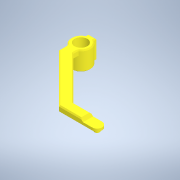
# Autodesk Inventor part: head_lock
Saved by Autodesk Inventor 2021 (Build 250183000, 183)
## iProperties
Created: 2021-02-04
Part Number: head_lock
Material: Generic
Document SubType Name: Modeling
Designer: Daniel
Density: 1 g/cm^3
Appearance: Default
Author: Daniel
Autodesk Inventor part; units mm, degrees
ref_plane "YZ Plane" through (0, 0, 0) normal (1, 0, 0) x (0, 1, 0)
ref_plane "XZ Plane" through (0, 0, 0) normal (0, 1, 0) x (-1, 0, 0)
ref_plane "XY Plane" through (0, 0, 0) normal (0, 0, 1) x (1, 0, 0)
sketch "Sketch1" plane through (0, 0, 0) normal (0, 1, 0) x (-1, 0, 0)
  arc A0 (-4.6069, -58.0567) -> (5, -60) centre (0, -60) ccw
  line L0 (0, 0) -> (-76, 0) construction
  line L1 (-5, -5) -> (-76, -5)
  line L2 (-76, 5) -> (5, 5)
  arc A1 (-76, 5) -> (-76, -5) centre (-76, 0) ccw
  circle A2 centre (0, -60) radius 2.25
  circle A3 centre (0, -60) radius 6.375
  circle A4 centre (0, -60) radius 11.375 construction
  line L3 (-5, -5) -> (-5, -52.0696)
  line L4 (5, 5) -> (5, -52.0696)
  circle A5 centre (0, -60) radius 9.375
  line L5 (-4, -68.4788) -> (4, -68.4788)
  line L6 (4, -68.4788) -> (4, -71.375)
  line L7 (4, -71.375) -> (-4, -71.375)
  line L8 (-4, -71.375) -> (-4, -68.4788)
  line L9 (0, -60) -> (0, -31.5447) construction
  line L10 (-47.4264, -5) -> (-5, -47.4264)
  line L11 (-43.2843, 5) -> (5, -43.2843)
  point P0 (-38, 0)
  point P1 (-8.5189, -5)
  point P2 (-5, -49.7828)
  point P3 (5, -49.7828)
  dimension "d9" = 4.5
  dimension "d24" = 5
  dimension "d29" = 12.75
  dimension "d30" = 5
  dimension "d46" = 76
  dimension "d49" = 10
  dimension "d50" = 6
  dimension "d51" = 3
  dimension "d53" = 8
  dimension "d55" = 60
  dimension "d56" = 5
  dimension "d58" = 90
  dimension "d59" = 10
  dimension "d60" = 10
  dimension "d61" = 45
  dimension "d62" = 30
  constraints: 26 end point, 8 parallel, 8 point on circle, 6 centre point, 5 coincident, 4 point on line, 3 tangent, 1 horizontal, 1 midpoint, 1 perpendicular, 1 vertical alignment
  measures "d9" diameter of A2
  measures "d24" radius of A0
  measures "d29" diameter of A3
  measures "d30" radial gap between concentric circles of A4 A3
  measures "d46" distance of L0.start L0.end
  measures "d49" distance between parallel lines of L4 L3
  measures "d50" distance of A0.start L3.end
  measures "d51" radial gap between concentric circles of A3 A5
  measures "d53" distance of L5.start L5.end
  measures "d55" distance of point (0, 0) A2.centre
  measures "d56" distance between parallel lines of L3 L9
  measures "d58" angle of L1 L3
  measures "d59" distance between parallel lines of L1 L2
  measures "d60" distance between parallel lines of L11 L10
  measures "d61" angle of L1 L10
  measures "d62" distance from line of L1.start L10
extrude "Extrusion1" add sketch "Sketch1" along normal blind 5 contours L1 A1 L2 L11 | L1 L11 L3 L10 | L3 L11 L4 A5 | A5 L5 | L5 A5 | A5 L6 L7 L8
sketch "Sketch2" plane through (0, 0, 0) normal (0, -1, 0) x (1, 0, 0)
  arc A0 (76, -5) -> (76, 5) centre (76, 0) ccw projected
  circle A1 centre (76, 0) radius 2.5
  point P0 (0, 0)
  dimension "d6" = 5
  constraints: 1 centre point, 1 coincident
  measures "d6" diameter of A1
extrude "Extrusion2" add sketch "Sketch2" along normal blind 3
sketch "Sketch4" plane through (-15.2896, 0, 5) normal (0, 0, 1) x (1, 0, 0)
  line L0 (96.2896, 0) -> (96.2896, 5) projected
  line L1 (96.2896, 2.5) -> (82.2896, 2.5)
  line L2 (82.2896, 2.5) -> (79.7896, 5)
  line L3 (79.7896, 5) -> (96.2896, 5)
  line L4 (96.2896, 2.5) -> (96.2896, 5)
  line L5 (58.5738, 5) -> (91.2896, 5) projected
  point P0 (15.2896, 0)
  point P1 (10.2896, 5)
  dimension "d17" = 135
  dimension "d19" = 14
  constraints: 8 end point, 2 collinear, 1 horizontal, 1 midpoint
  measures "d17" angle of L1 L2
  measures "d19" distance of L1.start L1.end
extrude "Extrusion4" cut sketch "Sketch4" against normal through all
sketch "Sketch7" plane through (0, 0, 0) normal (0, -1, 0) x (1, 0, 0)
  arc A0 (-0.8975, -50.6681) -> (6.2033, -52.9708) centre (0, -60) ccw
  circle A1 centre (0, -60) radius 6.4
  circle A2 centre (0, -60) radius 9.375
  arc A3 (-5, -52.0696) -> (-4, -68.4788) centre (0, -60) ccw projected
  circle A4 centre (76, 0) radius 2.5 projected
  line L0 (5, -47.4264) -> (5, -52.0696) projected
  line L1 (76, -5) -> (47.4264, -5) projected
  arc A5 (76, -5) -> (76, 5) centre (76, 0) ccw projected
  line L2 (43.2843, 5) -> (76, 5) projected
  line L3 (-5, -52.0696) -> (-5, -43.2843) projected
  arc A6 (-5, -52.0696) -> (-4, -68.4788) centre (0, -60) ccw projected
  line L4 (-4, -71.375) -> (-4, -68.4788) projected
  line L5 (4, -71.375) -> (-4, -71.375) projected
  line L6 (4, -68.4788) -> (4, -71.375) projected
  arc A7 (4, -68.4788) -> (5, -52.0696) centre (0, -60) ccw projected
  line L7 (47.4264, -5) -> (5, -47.4264) projected
  line L8 (-5, -43.2843) -> (43.2843, 5) projected
  point P0 (0, 0)
  dimension "d31" = 12.8
  constraints: 2 centre point, 2 coincident, 2 concentric, 2 point on circle, 3 other
  measures "d31" diameter of A1
extrude "Extrusion6" add sketch "Sketch7" along normal blind 14 contours A2 A0 | A0 L6 L5 L4
sketch "Sketch8" plane through (7.8055, 0, -71.375) normal (0, 0, 1) x (1, 0, 0)
  circle A0 centre (-7.8055, -6) radius 1.65
  line L0 (-17.1805, -14) -> (1.5695, -14) projected
  point P0 (-7.8055, 0)
  point P1 (-2.6893, 8)
  point P2 (-7.8055, -14)
  point P3 (-7.8055, -14)
  dimension "d34" = 3.3
  dimension "d47" = 8
  constraints: 2 vertical alignment, 1 centre point, 1 midpoint
  measures "d34" diameter of A0
  measures "d47" distance from line of L0 A0.centre
extrude "Extrusion7" cut sketch "Sketch8" along normal up to surface
fillet "Fillet2" radius 2 2 edges at (5, 2.5, -52.0696) (-5, 2.5, -52.0696)
chamfer "Chamfer1" distance 1 angle 45 13 edges at (53.8921, 5, 5) (55.9632, 5, -5) (5, 5, -49.2302) (5.2026, 5, -51.911) (9.3173, 5, -61.0388) (-5, 5, -47.1591) (-5.2026, 5, -51.911) (-9.3173, 5, -61.0388) (4, 5, -69.9269) (0, 5, -71.375) (-4, 5, -69.9269) (26.2132, 5, -26.2132) (19.1421, 5, -19.1421)
chamfer "Chamfer2" distance 1 angle 45 5 edges at (-6.4, -14, -60) (0, -14, -50.625) (4, -14, -69.9269) (0, -14, -71.375) (-4, -14, -69.9269)
equation "\"d56\" = 0.5 * d49"
equation "\"d60\" = d49"
equation "\"d4\" = d24"
body "Solid1"
